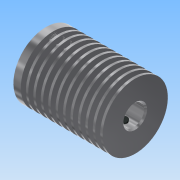
# Autodesk Inventor part: рАДИАТОР Е3DV6
Saved by Autodesk Inventor 2017 (Build 210142000, 142)
## iProperties
Part Number: рАДИАТОР Е3DV6
Material: Типовые
Document SubType Name: Modeling
Designer: Max
Mass: 5.64212 g
Surface Area: 90.0327 cm^2
Volume: 5.64212 cm^3
Density: 1 g/cm^3
Appearance: Алюминий — полированный
Author: Max
Autodesk Inventor part; units mm, degrees
ref_plane "YZ Plane" through (0, 0, 0) normal (1, 0, 0) x (0, 1, 0)
ref_plane "XZ Plane" through (0, 0, 0) normal (0, 1, 0) x (-1, 0, 0)
ref_plane "XY Plane" through (0, 0, 0) normal (0, 0, 1) x (1, 0, 0)
sketch "Эскиз1" plane through (0, 0, 0) normal (0, 1, 0) x (-1, 0, 0)
  line L0 (0, 0) -> (51.5187, 0) construction
  line L1 (0, 0) -> (0, 10.95)
  line L2 (0, 3.5) -> (15.13, 3.5)
  line L3 (15.13, 3.5) -> (15.13, 2.1)
  line L4 (15.13, 2.1) -> (21.4, 2.1)
  line L5 (0, 3.5) -> (0, 10.95)
  line L6 (0, 10.95) -> (0.82, 10.95)
  line L7 (0.82, 10.95) -> (0.82, 6.65)
  line L8 (0.82, 6.65) -> (2.52, 6.65)
  line L9 (2.52, 6.65) -> (2.52, 10.95)
  line L10 (2.52, 10.95) -> (3.32, 10.95)
  line L11 (3.32, 10.95) -> (3.32, 6.65)
  line L12 (5.82, 10.95) -> (5.82, 6.65)
  line L13 (5.02, 10.95) -> (5.82, 10.95)
  line L14 (5.02, 6.65) -> (5.02, 10.95)
  line L15 (3.32, 6.65) -> (5.02, 6.65)
  line L16 (8.32, 10.95) -> (8.32, 6.65)
  line L17 (7.52, 10.95) -> (8.32, 10.95)
  line L18 (7.52, 6.65) -> (7.52, 10.95)
  line L19 (5.82, 6.65) -> (7.52, 6.65)
  line L20 (10.82, 10.95) -> (10.82, 6.65)
  line L21 (10.02, 10.95) -> (10.82, 10.95)
  line L22 (10.02, 6.65) -> (10.02, 10.95)
  line L23 (8.32, 6.65) -> (10.02, 6.65)
  line L24 (13.32, 10.95) -> (13.32, 6.65)
  line L25 (12.52, 10.95) -> (13.32, 10.95)
  line L26 (12.52, 6.65) -> (12.52, 10.95)
  line L27 (10.82, 6.65) -> (12.52, 6.65)
  line L28 (15.82, 10.95) -> (15.82, 6.65)
  line L29 (15.02, 10.95) -> (15.82, 10.95)
  line L30 (15.02, 6.65) -> (15.02, 10.95)
  line L31 (13.32, 6.65) -> (15.02, 6.65)
  line L32 (18.32, 10.95) -> (18.32, 6.65)
  line L33 (17.52, 10.95) -> (18.32, 10.95)
  line L34 (17.52, 6.65) -> (17.52, 10.95)
  line L35 (15.82, 6.65) -> (17.52, 6.65)
  line L36 (20.82, 10.95) -> (20.82, 6.65)
  line L37 (20.02, 10.95) -> (20.82, 10.95)
  line L38 (20.02, 6.65) -> (20.02, 10.95)
  line L39 (18.32, 6.65) -> (20.02, 6.65)
  line L40 (23.32, 10.95) -> (23.32, 6.65)
  line L41 (22.52, 10.95) -> (23.32, 10.95)
  line L42 (22.52, 6.65) -> (22.52, 10.95)
  line L43 (20.82, 6.65) -> (22.52, 6.65)
  line L44 (25.82, 10.95) -> (25.82, 6.65)
  line L45 (25.02, 10.95) -> (25.82, 10.95)
  line L46 (25.02, 6.65) -> (25.02, 10.95)
  line L47 (23.32, 6.65) -> (25.02, 6.65)
  line L48 (25.82, 6.65) -> (27.52, 6.65)
  line L49 (27.52, 6.65) -> (27.52, 10.95)
  line L50 (27.52, 10.95) -> (30, 10.95)
  line L51 (30, 10.95) -> (30, 0)
  line L52 (30, 4.5) -> (21.4, 4.5)
  line L53 (21.4, 4.5) -> (21.4, 2.1)
  line L54 (23.32, 0) -> (30, 0)
  line L55 (30, 0) -> (30, 4.5)
  dimension "d0" = 3.5
  dimension "d1" = 2.1
  dimension "d2" = 15.13
  dimension "d3" = 4.3
  dimension "d4" = 10.95
  dimension "d5" = 0.82
  dimension "d6" = 1.7
  dimension "d7" = 0.8
  dimension "d16" = 30
  dimension "d18" = 2.48
  dimension "d19" = 1.7
  dimension "d20" = 4.5
  dimension "d21" = 8.6
  constraints: 112 end point, 16 point on line, 9 perpendicular, 5 horizontal, 3 parallel, 1 collinear, 1 vertical
  measures "d0" distance between parallel lines of L0 L2
  measures "d1" distance between parallel lines of L0 L4
  measures "d2" distance between parallel lines of L1 L3
  measures "d3" distance between parallel lines of L8 L6
  measures "d4" distance between parallel lines of L6 L0
  measures "d5" distance between parallel lines of L1 L7
  measures "d6" distance between parallel lines of L7 L9
  measures "d7" distance between parallel lines of L9 L11
  measures "d16" distance between parallel lines of L1 L51
  measures "d18" distance between parallel lines of L49 L51
  measures "d19" distance between parallel lines of L44 L49
  measures "d20" distance between parallel lines of L0 L52
  measures "d21" distance between parallel lines of L53 L51
revolve "Вращение1" add sketch "Эскиз1" angle 360 about axis through (0, 0, 0) along (-1, 0, 0)
chamfer "Фаска1" distance 1 angle 45 1 edges at (-21.4, 0, -2.1)
thread "Резьба1" size "M9x1.25" class "6H" standard "ANSI Metric M Profile" full length
sketch "Эскиз3" plane through (-30, 0, 0) normal (0, 1, 0) x (0, 0, 1)
  line L0 (4.5, 0) -> (4.5, 8.6)
  line L1 (4.5, 8.6) -> (3.5732, 8.6)
  line L2 (3.5732, 8.6) -> (3.5732, 0)
  line L3 (3.5732, 0) -> (4.5, 0)
  line L4 (0, -1.72) -> (0, 10.32) projected
  constraints: 8 end point
revolve "Вращение2" add sketch "Эскиз3" angle 360 about axis through (-30, 0, 0) along (1, 0, 0) separate body
sketch "Эскиз2" plane through (-30, 0, 4.5) normal (0, -1, 0) x (1, 0, 0)
  line L0 (-0.7293, -0.0634) -> (-0.6251, -0.0634) construction
  line L1 (0.1041, -0.8638) -> (-0.0001, -1.0639) construction
  line L2 (-1.2501, -1.0639) -> (-1.3543, -0.8638) construction
  line L3 (-0.5209, -0.0634) -> (-0.6251, 0.1367) construction
  line L4 (-0.6251, 0.1367) -> (-0.7293, -0.0634) construction
  line L5 (-1.2501, -1.0639) -> (-1.1459, -0.8638) construction
  line L6 (-0.5209, -0.0634) -> (-0.1043, -0.8638)
  line L7 (-1.3543, -0.8638) -> (-1.1459, -0.8638) construction
  arc A0 (-1.3543, -0.8638) -> (-1.2501, -0.927) centre (-1.2501, -0.8096) ccw construction
  line L8 (0.1041, -0.8638) -> (-0.1043, -0.8638) construction
  line L9 (-1.2501, -1.0639) -> (-1.2501, -0.8638) construction
  line L10 (-0.0001, -1.0639) -> (-0.0001, -0.8638) construction
  line L11 (-0.6251, 0.1367) -> (-0.6251, -0.0002) construction
  line L12 (-1.2501, -0.927) -> (-0.0001, -0.927)
  arc A1 (-1.2501, -0.927) -> (-1.1459, -0.8638) centre (-1.2501, -0.8096) ccw
  line L13 (-0.1043, -0.8638) -> (-0.0001, -1.0639) construction
  line L14 (-1.1459, -0.8638) -> (-0.7293, -0.0634)
  line L15 (-0.0001, -0.0002) -> (-0.0001, 0.0177)
  line L16 (-0.0001, 0.0177) -> (-0.0001, -0.0002)
  line L17 (-0.0001, -0.0002) -> (0.0334, -0.0002)
  arc A2 (-0.1043, -0.8638) -> (-0.0001, -0.927) centre (-0.0001, -0.8096) ccw
  arc A3 (-0.0001, -0.927) -> (0.1041, -0.8638) centre (-0.0001, -0.8096) ccw construction
  arc A4 (-0.6251, -0.0002) -> (-0.7293, -0.0634) centre (-0.6251, -0.1176) ccw
  arc A5 (-0.5209, -0.0634) -> (-0.6251, -0.0002) centre (-0.6251, -0.1176) ccw
  line L18 (-0.6251, -0.0002) -> (-0.6251, -0.0634) construction
  line L19 (-0.6251, -0.0634) -> (-0.5209, -0.0634) construction
  dimension "d28" = 55
  dimension "d29" = 0.2001
  dimension "d30" = 0.2001
  dimension "Эскиз2_ThreadOffset" = 0
  dimension "Эскиз2_MajorRadius" = 0.9268
  dimension "d33" = 1.25
  dimension "Эскиз2_MinorRadius" = 0
  constraints: 40 end point, 12 point on circle, 10 parallel, 8 tangent, 6 centre point, 6 collinear, 2 midpoint, 2 point on line, 1 horizontal, 1 perpendicular, 3 other
  measures "d28" angle of L6 L14
  measures "d29" distance of L3.end L0.end
  measures "d30" distance of L1.end L10.end
  measures "Эскиз2_ThreadOffset" distance between parallel lines of L15 L10
  measures "Эскиз2_MajorRadius" distance from line of L12 L15.start
  measures "d33" distance from line of L1.end L9
  measures "Эскиз2_MinorRadius" distance edge to line of A5 L17
coil "Пружина1" sketch "Эскиз2" operation cut axis through (-30, 0, 0) along (1, 0, 0) pitch 1.2513 turns 8.871129 hand right bodies 2
chamfer "Фаска2" distance 0.5 angle 45 1 edges at (0, 0, -3.5)
sketch "Эскиз4" plane through (0, 0, 0) normal (0, 0, 1) x (1, 0, 0)
  line L0 (0, 0) -> (-34.4606, 0) construction
  circle A0 centre (-4.2, 0) radius 1.5
  circle A1 centre (-11.5, 0) radius 1.5
  line L1 (0, 10.95) -> (0, -10.95) projected
  line L2 (-12.366, 0) -> (-11.933, 0.75)
  line L3 (-11.933, 0.75) -> (-11.067, 0.75)
  line L4 (-11.067, 0.75) -> (-10.634, 0)
  line L5 (-10.634, 0) -> (-11.067, -0.75)
  line L6 (-11.067, -0.75) -> (-11.933, -0.75)
  line L7 (-11.933, -0.75) -> (-12.366, 0)
  line L8 (-5.066, 0) -> (-4.633, 0.75)
  line L9 (-4.633, 0.75) -> (-3.767, 0.75)
  line L10 (-3.767, 0.75) -> (-3.334, 0)
  line L11 (-3.334, 0) -> (-3.767, -0.75)
  line L12 (-3.767, -0.75) -> (-4.633, -0.75)
  line L13 (-4.633, -0.75) -> (-5.066, 0)
  dimension "d49" = 3
  dimension "d50" = 3
  dimension "d51" = 7.3
  dimension "d52" = 4.2
  dimension "d55" = 1.5
  dimension "d56" = 1.5
  constraints: 26 end point, 4 point on line, 2 centre point, 2 coincident, 1 horizontal, 26 other
  measures "d49" diameter of A0
  measures "d50" diameter of A1
  measures "d51" distance of A0.centre A1.centre
  measures "d52" distance from line of L1 A0.centre
  measures "d55" distance between parallel lines of L6 L3
  measures "d56" distance between parallel lines of L12 L9
extrude "Выдавливание1" cut sketch "Эскиз4" against normal blind 30 contours A0 | A1 | L2 L3 L4 L5 L6 L7 | L8 L9 L10 L11 L12 L13 bodies 1
extrude "Выдавливание2" add sketch "Эскиз4" against normal blind 5 bodies 1
extrude "Выдавливание3" add sketch "Эскиз4" against normal blind 4 contours L2 L3 L4 L5 L6 L7 | L8 L9 L10 L11 L12 L13 bodies 1
extrude "Выдавливание4" cut sketch "Эскиз4" against normal blind 3 contours A0 | A1 | L2 L3 L4 L5 L6 L7 | L8 L9 L10 L11 L12 L13 bodies 1
sketch "Эскиз5" plane through (-30, 0, 0) normal (-1, 0, 0) x (0, 0, 1)
  circle A0 centre (9, 0) radius 1.5
  circle A1 centre (-9, 0) radius 1.5
  line L0 (0, 0) -> (0, -5.2607) construction
  dimension "d63" = 3
  dimension "d64" = 3
  dimension "d65" = 18
  constraints: 2 centre point, 2 end point, 1 symmetric about line, 1 vertical
  measures "d63" diameter of A0
  measures "d64" diameter of A1
  measures "d65" distance of A0.centre A1.centre
extrude "Выдавливание5" cut sketch "Эскиз5" against normal blind 7.6 bodies 1
thread "Резьба2" size "M3x0.5" class "6H" standard "ANSI Metric M Profile" full length
thread "Резьба3" size "M3x0.5" class "6H" standard "ANSI Metric M Profile" full length
sketch "Эскиз7" plane through (-27.52, 0, 9) normal (0, -1, 0) x (0, 0, 1)
  line L0 (1.5, 0) -> (1.5, 2.48)
  line L1 (1.5, 2.48) -> (1.1293, 2.48)
  line L2 (1.1293, 2.48) -> (1.1293, 0)
  line L3 (1.1293, 0) -> (1.5, 0)
  line L4 (0, -0.496) -> (0, 2.976) projected
  constraints: 8 end point
revolve "Вращение3" add sketch "Эскиз7" angle 360 about axis through (-27.52, 0, 9) along (-1, 0, 0) separate body
sketch "Эскиз6" plane through (-27.52, 0, 10.5) normal (0, 1, 0) x (-1, 0, 0)
  line L0 (-0.2918, -0.0255) -> (-0.2501, -0.0255) construction
  line L1 (0.0416, -0.3456) -> (-0.0001, -0.4257) construction
  line L2 (-0.5001, -0.4257) -> (-0.5418, -0.3456) construction
  line L3 (-0.2084, -0.0255) -> (-0.2501, 0.0546) construction
  line L4 (-0.2501, 0.0546) -> (-0.2918, -0.0255) construction
  line L5 (-0.5001, -0.4257) -> (-0.4584, -0.3456) construction
  line L6 (-0.2084, -0.0255) -> (-0.0418, -0.3456)
  line L7 (-0.5418, -0.3456) -> (-0.4584, -0.3456) construction
  arc A0 (-0.5418, -0.3456) -> (-0.5001, -0.3709) centre (-0.5001, -0.3239) ccw construction
  line L8 (0.0416, -0.3456) -> (-0.0418, -0.3456) construction
  line L9 (-0.5001, -0.4257) -> (-0.5001, -0.3456) construction
  line L10 (-0.0001, -0.4257) -> (-0.0001, -0.3456) construction
  line L11 (-0.2501, 0.0546) -> (-0.2501, -0.0002) construction
  line L12 (-0.5001, -0.3709) -> (-0.0001, -0.3709)
  arc A1 (-0.5001, -0.3709) -> (-0.4584, -0.3456) centre (-0.5001, -0.3239) ccw
  line L13 (-0.0418, -0.3456) -> (-0.0001, -0.4257) construction
  line L14 (-0.4584, -0.3456) -> (-0.2918, -0.0255)
  line L15 (-0.0001, -0.0002) -> (-0.0001, 0.0177)
  line L16 (-0.0001, 0.0177) -> (-0.0001, -0.0002)
  line L17 (-0.0001, -0.0002) -> (0.0334, -0.0002)
  arc A2 (-0.0418, -0.3456) -> (-0.0001, -0.3709) centre (-0.0001, -0.3239) ccw
  arc A3 (-0.0001, -0.3709) -> (0.0416, -0.3456) centre (-0.0001, -0.3239) ccw construction
  arc A4 (-0.2501, -0.0002) -> (-0.2918, -0.0255) centre (-0.2501, -0.0471) ccw
  arc A5 (-0.2084, -0.0255) -> (-0.2501, -0.0002) centre (-0.2501, -0.0471) ccw
  line L18 (-0.2501, -0.0002) -> (-0.2501, -0.0255) construction
  line L19 (-0.2501, -0.0255) -> (-0.2084, -0.0255) construction
  dimension "d72" = 55
  dimension "d73" = 0.08
  dimension "d74" = 0.08
  dimension "Эскиз6_ThreadOffset" = 0
  dimension "Эскиз6_MajorRadius" = 0.3707
  dimension "d77" = 0.5
  dimension "Эскиз6_MinorRadius" = 0
  constraints: 40 end point, 12 point on circle, 10 parallel, 8 tangent, 6 centre point, 6 collinear, 2 midpoint, 2 point on line, 1 horizontal, 1 perpendicular, 3 other
  measures "d72" angle of L6 L14
  measures "d73" distance of L3.end L0.end
  measures "d74" distance of L1.end L10.end
  measures "Эскиз6_ThreadOffset" distance between parallel lines of L15 L10
  measures "Эскиз6_MajorRadius" distance from line of L12 L15.start
  measures "d77" distance from line of L1.end L9
  measures "Эскиз6_MinorRadius" distance edge to line of A5 L17
coil "Пружина2" sketch "Эскиз6" operation cut axis through (-27.52, 0, 9) along (-1, 0, 0) pitch 0.5005 turns 6.953047 hand right bodies 3
sketch "Эскиз9" plane through (-27.52, 0, -9) normal (0, -1, 0) x (0, 0, 1)
  line L0 (1.5, 0) -> (1.5, 2.48)
  line L1 (1.5, 2.48) -> (1.1293, 2.48)
  line L2 (1.1293, 2.48) -> (1.1293, 0)
  line L3 (1.1293, 0) -> (1.5, 0)
  line L4 (0, -0.496) -> (0, 2.976) projected
  constraints: 8 end point
revolve "Вращение4" add sketch "Эскиз9" angle 360 about axis through (-27.52, 0, -9) along (-1, 0, 0) separate body
sketch "Эскиз8" plane through (-27.52, 0, -7.5) normal (0, 1, 0) x (-1, 0, 0)
  line L0 (-0.2918, -0.0255) -> (-0.2501, -0.0255) construction
  line L1 (0.0416, -0.3456) -> (-0.0001, -0.4257) construction
  line L2 (-0.5001, -0.4257) -> (-0.5418, -0.3456) construction
  line L3 (-0.2084, -0.0255) -> (-0.2501, 0.0546) construction
  line L4 (-0.2501, 0.0546) -> (-0.2918, -0.0255) construction
  line L5 (-0.5001, -0.4257) -> (-0.4584, -0.3456) construction
  line L6 (-0.2084, -0.0255) -> (-0.0418, -0.3456)
  line L7 (-0.5418, -0.3456) -> (-0.4584, -0.3456) construction
  arc A0 (-0.5418, -0.3456) -> (-0.5001, -0.3709) centre (-0.5001, -0.3239) ccw construction
  line L8 (0.0416, -0.3456) -> (-0.0418, -0.3456) construction
  line L9 (-0.5001, -0.4257) -> (-0.5001, -0.3456) construction
  line L10 (-0.0001, -0.4257) -> (-0.0001, -0.3456) construction
  line L11 (-0.2501, 0.0546) -> (-0.2501, -0.0002) construction
  line L12 (-0.5001, -0.3709) -> (-0.0001, -0.3709)
  arc A1 (-0.5001, -0.3709) -> (-0.4584, -0.3456) centre (-0.5001, -0.3239) ccw
  line L13 (-0.0418, -0.3456) -> (-0.0001, -0.4257) construction
  line L14 (-0.4584, -0.3456) -> (-0.2918, -0.0255)
  line L15 (-0.0001, -0.0002) -> (-0.0001, 0.0177)
  line L16 (-0.0001, 0.0177) -> (-0.0001, -0.0002)
  line L17 (-0.0001, -0.0002) -> (0.0334, -0.0002)
  arc A2 (-0.0418, -0.3456) -> (-0.0001, -0.3709) centre (-0.0001, -0.3239) ccw
  arc A3 (-0.0001, -0.3709) -> (0.0416, -0.3456) centre (-0.0001, -0.3239) ccw construction
  arc A4 (-0.2501, -0.0002) -> (-0.2918, -0.0255) centre (-0.2501, -0.0471) ccw
  arc A5 (-0.2084, -0.0255) -> (-0.2501, -0.0002) centre (-0.2501, -0.0471) ccw
  line L18 (-0.2501, -0.0002) -> (-0.2501, -0.0255) construction
  line L19 (-0.2501, -0.0255) -> (-0.2084, -0.0255) construction
  dimension "d90" = 55
  dimension "d91" = 0.08
  dimension "d92" = 0.08
  dimension "Эскиз8_ThreadOffset" = 0
  dimension "Эскиз8_MajorRadius" = 0.3707
  dimension "d95" = 0.5
  dimension "Эскиз8_MinorRadius" = 0
  constraints: 40 end point, 12 point on circle, 10 parallel, 8 tangent, 6 centre point, 6 collinear, 2 midpoint, 2 point on line, 1 horizontal, 1 perpendicular, 3 other
  measures "d90" angle of L6 L14
  measures "d91" distance of L3.end L0.end
  measures "d92" distance of L1.end L10.end
  measures "Эскиз8_ThreadOffset" distance between parallel lines of L15 L10
  measures "Эскиз8_MajorRadius" distance from line of L12 L15.start
  measures "d95" distance from line of L1.end L9
  measures "Эскиз8_MinorRadius" distance edge to line of A5 L17
coil "Пружина3" sketch "Эскиз8" operation cut axis through (-27.52, 0, -9) along (-1, 0, 0) pitch 0.5005 turns 6.953047 hand right bodies 4
equation "\"d28\" = d35"
equation "\"d29\" = 0.160083 * Эскиз2_Pitch"
equation "\"d30\" = 0.160083 * Эскиз2_Pitch"
equation "\"d33\" = Эскиз2_Pitch"
equation "\"d72\" = d79"
equation "\"d73\" = 0.160083 * Эскиз6_Pitch"
equation "\"d74\" = 0.160083 * Эскиз6_Pitch"
equation "\"d77\" = Эскиз6_Pitch"
equation "\"d90\" = d97"
equation "\"d91\" = 0.160083 * Эскиз8_Pitch"
equation "\"d92\" = 0.160083 * Эскиз8_Pitch"
equation "\"d95\" = Эскиз8_Pitch"
equation "\"d35\" = 55deg"
equation "\"Эскиз2_Pitch\" = 1.25"
equation "\"d79\" = 55deg"
equation "\"Эскиз6_Pitch\" = 0.5"
equation "\"d97\" = 55deg"
equation "\"Эскиз8_Pitch\" = 0.5"
